Autodesk Inventor part; units mm, degrees
(part 2 of 2)
sketch "Skizze59" plane through (0, 0, -3.6) normal (0, 0, -1) x (-1, 0, 0)
  line L0 (-0.896059, 8.16056) -> (-0.896059, 11.335987)
  line L1 (1.853941, 6.572847) -> (-0.896059, 8.16056)
  line L2 (4.603941, 8.16056) -> (1.853941, 6.572847)
  line L3 (4.603941, 11.335987) -> (4.603941, 8.16056)
  line L4 (1.853941, 12.9237) -> (4.603941, 11.335987)
  line L5 (-0.896059, 11.335987) -> (1.853941, 12.9237)
  circle A0 centre (1.853941, 9.748273) radius 1.6
  line L6 (-11.645804, 4.46348) -> (-8.470378, 4.46348)
  line L7 (-13.233518, 1.71348) -> (-11.645804, 4.46348)
  line L8 (-11.645804, -1.03652) -> (-13.233518, 1.71348)
  line L9 (-8.470378, -1.03652) -> (-11.645804, -1.03652)
  line L10 (-6.882665, 1.71348) -> (-8.470378, -1.03652)
  line L11 (-8.470378, 4.46348) -> (-6.882665, 1.71348)
  circle A1 centre (-10.058091, 1.71348) radius 1.6
  line L12 (8.300321, 0.586285) -> (11.475747, 0.586285)
  line L13 (6.712608, -2.163715) -> (8.300321, 0.586285)
  line L14 (8.300321, -4.913715) -> (6.712608, -2.163715)
  line L15 (11.475747, -4.913715) -> (8.300321, -4.913715)
  line L16 (13.063461, -2.163715) -> (11.475747, -4.913715)
  line L17 (11.475747, 0.586285) -> (13.063461, -2.163715)
  circle A2 centre (9.888034, -2.163715) radius 1.6
  line L18 (-3.611084, -7.448215) -> (-0.435657, -7.448215)
  line L19 (-5.198797, -10.198215) -> (-3.611084, -7.448215)
  line L20 (-3.611084, -12.948215) -> (-5.198797, -10.198215)
  line L21 (-0.435657, -12.948215) -> (-3.611084, -12.948215)
  line L22 (1.152056, -10.198215) -> (-0.435657, -12.948215)
  line L23 (-0.435657, -7.448215) -> (1.152056, -10.198215)
  circle A3 centre (-2.023371, -10.198215) radius 1.6
  point P0 (0, 0)
extrude "Extrusion44" cut sketch "Skizze55" against normal blind 4.4 contours L0 L1 L2 L3 L4 L5 | L6 L7 L8 L9 L10 L11 | L12 L13 L14 L15 L16 L17 | L18 L19 L20 L21 L22 L23
sketch "Skizze60" plane through (0, 0, -6) normal (0, 0, -1) x (-1, 0, 0)
  circle A0 centre (-10.058091, 1.71348) radius 1.6
  line L0 (-8.470378, -1.03652) -> (-11.645804, -1.03652)
  line L1 (-6.882665, 1.71348) -> (-8.470378, -1.03652)
  line L2 (-8.470378, 4.46348) -> (-6.882665, 1.71348)
  line L3 (-11.645804, 4.46348) -> (-8.470378, 4.46348)
  line L4 (-13.233518, 1.71348) -> (-11.645804, 4.46348)
  line L5 (-11.645804, -1.03652) -> (-13.233518, 1.71348)
  circle A1 centre (1.853941, 9.748273) radius 1.6
  line L6 (4.603941, 11.335987) -> (4.603941, 8.16056)
  line L7 (1.853941, 12.9237) -> (4.603941, 11.335987)
  line L8 (-0.896059, 11.335987) -> (1.853941, 12.9237)
  line L9 (-0.896059, 8.16056) -> (-0.896059, 11.335987)
  line L10 (1.853941, 6.572847) -> (-0.896059, 8.16056)
  line L11 (4.603941, 8.16056) -> (1.853941, 6.572847)
  circle A2 centre (9.888034, -2.163715) radius 1.6
  line L12 (11.475747, -4.913715) -> (8.300321, -4.913715)
  line L13 (13.063461, -2.163715) -> (11.475747, -4.913715)
  line L14 (11.475747, 0.586285) -> (13.063461, -2.163715)
  line L15 (8.300321, 0.586285) -> (11.475747, 0.586285)
  line L16 (6.712608, -2.163715) -> (8.300321, 0.586285)
  line L17 (8.300321, -4.913715) -> (6.712608, -2.163715)
  circle A3 centre (-2.023371, -10.198215) radius 1.6
  line L18 (-0.435657, -12.948215) -> (-3.611084, -12.948215)
  line L19 (1.152056, -10.198215) -> (-0.435657, -12.948215)
  line L20 (-0.435657, -7.448215) -> (1.152056, -10.198215)
  line L21 (-3.611084, -7.448215) -> (-0.435657, -7.448215)
  line L22 (-5.198797, -10.198215) -> (-3.611084, -7.448215)
  line L23 (-3.611084, -12.948215) -> (-5.198797, -10.198215)
  point P0 (0, 0)
extrude "Extrusion45" add sketch "Skizze60" against normal blind 2
sketch "Skizze61" plane through (0, 0, -6) normal (0, 0, -1) x (-1, 0, 0)
  point P0 (0, 0)
sketch "Skizze62" plane through (0, 0, 0) normal (0, 0, 1) x (1, 0, 0)
  circle A0 centre (0, 0) radius 17.5
  circle A1 centre (0, 0) radius 4
  circle A2 centre (-1.853941, 9.748273) radius 1.6
  circle A3 centre (2.023371, -10.198215) radius 1.6
  circle A4 centre (-9.888034, -2.163715) radius 1.6
  circle A5 centre (10.058091, 1.71348) radius 1.6
extrude "Extrusion46" add sketch "Skizze62" along normal blind 3
sketch "Skizze63" plane through (0, 0, -6) normal (0, 0, -1) x (-1, 0, 0)
  circle A0 centre (0, 0) radius 15.278
  circle A1 centre (0, 13.758053) radius 3
  dimension "d220" = 6
  constraints: 1 centre point
  measures "d220" diameter of A1
sketch "Skizze64" plane through (0, 0, -6) normal (0, 0, -1) x (-1, 0, 0)
  circle A0 centre (1.853941, 9.748273) radius 1.6
  circle A1 centre (-10.058091, 1.71348) radius 1.6
  circle A2 centre (-2.023371, -10.198215) radius 1.6
  circle A3 centre (9.888034, -2.163715) radius 1.6
  point P0 (0, 0)
extrude "Extrusion47" add sketch "Skizze64" against normal blind 2
extrude "Extrusion48" cut sketch "Skizze63" against normal blind 1.5 contours A1 A0 | A0 A1 picked at (-0.100274, 13.75834) picked at (0, 15.753299)
pattern_circular "Runde Anordnung1" count 10 over 360 about axis through (0, 0, -10) along (0, 0, 1) of "Extrusion48"
sketch "Skizze65" plane through (0, 0, -6) normal (0, 0, -1) x (-1, 0, 0)
  circle A0 centre (0, 13.758053) radius 3
  circle A1 centre (0, 0) radius 13.758053
  circle A2 centre (0, 0) radius 11.258
  circle A3 centre (0, 0) radius 16.258
  point P0 (2.694238, 12.438554)
  point P1 (-0.896059, 10.895)
  dimension "d229" = 22.516
  dimension "d230" = 32.516
  constraints: 3 coincident, 2 centre point, 1 vertical alignment, 2 other
  measures "d229" diameter of A2
  measures "d230" diameter of A3
extrude "Extrusion49" cut sketch "Skizze65" against normal blind 1 contours A0 A1 A3 | A0 A3 A1 | A1 A0 A2 | A0 A2 A1
sketch "Skizze66" plane through (0, -13.758053, -4.5) normal (0, 0, -1) x (-1, 0, 0)
  arc A0 (1.496689, 2.599985) -> (-1.496689, 2.599985) centre (0, 0) ccw
  circle A1 centre (0, 0) radius 3
  circle A2 centre (0, 0) radius 1.25
  circle A3 centre (0, 0) radius 3
  point P0 (0, 13.758053)
  point P1 (-1.496689, 2.599985)
  point P2 (1.496689, 2.599985)
  dimension "d237" = 2.5
  constraints: 3 centre point, 3 coincident
  measures "d237" diameter of A2
extrude "Extrusion50" add sketch "Skizze66" along normal up to surface (0.5 mm away)
pattern_circular "Runde Anordnung3" count 10 over 360 about axis through (0, 0, -10) along (0, 0, 1) of "Extrusion50"
sketch "Skizze67" plane through (0, 0, -6) normal (0, 0, -1) x (-1, 0, 0)
  circle A0 centre (0, -13.758053) radius 1.25
  circle A1 centre (0, -13.758053) radius 1.25
  arc A2 (1.496689, -11.158068) -> (-1.496689, -11.158068) centre (0, -13.758053) ccw
  circle A3 centre (0, -13.758053) radius 3
  point P0 (0, 0)
  point P1 (-1.496689, -11.158068)
  point P2 (1.496689, -11.158068)
  constraints: 2 centre point, 2 coincident
extrude "Extrusion51" cut sketch "Skizze67" against normal up to surface (1 mm away)
pattern_circular "Runde Anordnung4" count 20 over 360 about axis through (0, 0, -10) along (0, 0, 1) of "Extrusion51"
sketch "Skizze68" plane through (0, 0, -6) normal (0, 0, -1) x (-1, 0, 0)
  circle A0 centre (0, -13.758053) radius 1.25
  circle A1 centre (0, -13.758053) radius 1.25
  point P0 (0, 0)
  constraints: 1 centre point, 1 coincident
extrude "Extrusion52" cut sketch "Skizze68" against normal up to surface (1.5 mm away)
pattern_circular "Runde Anordnung5" count 20 over 360 about axis through (0, 0, -10) along (0, 0, 1) of "Extrusion52"
fillet "Rundung9" radius 0.5 1 edges at (12.6984, 5.4403, -5)
pattern_circular "Runde Anordnung6" count 20 over 360 about axis through (0, 0, -10) along (0, 0, 1) of "Rundung9"
sketch "Skizze69" plane through (0, 0, -6) normal (0, 0, -1) x (-1, 0, 0)
  point P0 (0, 0)
